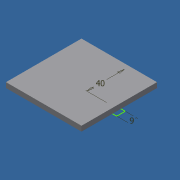
# Autodesk Inventor part: HotendMountCarriage
Saved by Autodesk Inventor 2018 (Build 220112000, 112)
## iProperties
Created: 2022-08-29
Part Number: HotendMountCarriage
Material: Generic
Document SubType Name: Modeling
Designer: Nathann
Density: 1 g/cm^3
Appearance: Default
Author: Nathann
Autodesk Inventor part; units mm, degrees
ref_plane "YZ Plane" through (0, 0, 0) normal (1, 0, 0) x (0, 1, 0)
ref_plane "XZ Plane" through (0, 0, 0) normal (0, 1, 0) x (-1, 0, 0)
ref_plane "XY Plane" through (0, 0, 0) normal (0, 0, 1) x (1, 0, 0)
sketch "Sketch1" plane through (0, 0, 0) normal (0, 0, 1) x (1, 0, 0)
  line L0 (0, 0) -> (80, 0)
  line L1 (80, 0) -> (80, -80)
  line L2 (80, -80) -> (0, -80)
  line L3 (0, -80) -> (0, 0)
  dimension "d0" = 80
  dimension "d1" = 80
  constraints: 8 end point, 2 parallel, 1 horizontal, 1 perpendicular
  measures "d0" distance of L0.start L0.end
  measures "d1" distance of L2.end L0.start
extrude "Extrusion1" add sketch "Sketch1" along normal blind 5.4
sketch "Sketch2" plane through (0, 0, 0) normal (0, 0, -1) x (-1, 0, 0)
  circle A0 centre (-67.059, -40) radius 7.1216
  line L0 (-60.1896, -38.1216) -> (-84.2475, -38.1216)
  line L1 (-84.2475, -38.1216) -> (-84.2475, -47.1216)
  line L2 (-84.2475, -47.1216) -> (-60.1896, -47.1216)
  line L3 (-60.1896, -47.1216) -> (-60.1896, -38.1216)
  line L4 (0, 0) -> (-80, 0) projected
  dimension "d4" = 40
  dimension "d6" = 9
  constraints: 8 end point, 2 horizontal, 2 parallel, 1 perpendicular, 3 other
  measures "d4" distance from line of L4 point (-67.059, -40)
  measures "d6" distance of L0.end L1.end
equation "\"RodDiameter\" = 8"
equation "\"VerticalBearingOD\" = 16"
equation "\"PrintingClearance\" = 0.2"
body "Solid1"
